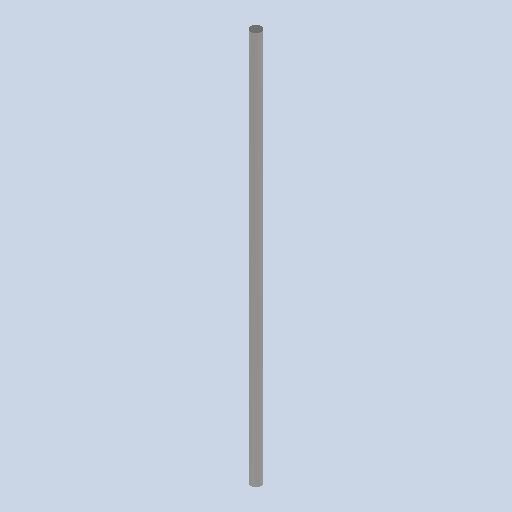
# Autodesk Inventor part: Axis
Saved by Autodesk Inventor 2023 (Build 270158000, 158)
## iProperties
Created: 2023-02-18
Part Number: Axis
Material: Stainless Steel
Document SubType Name: Modeling
Designer: phill
Density: 8 g/cm^3
Appearance: Semi-Polished
Author: phill
Autodesk Inventor part; units mm, degrees
ref_plane "YZ Plane" through (0, 0, 0) normal (1, 0, 0) x (0, 1, 0)
ref_plane "XZ Plane" through (0, 0, 0) normal (0, 1, 0) x (-1, 0, 0)
ref_plane "XY Plane" through (0, 0, 0) normal (0, 0, 1) x (1, 0, 0)
sketch "Sketch1" plane through (0, 0, 0) normal (0, 1, 0) x (-1, 0, 0)
  circle A0 centre (0, -107) radius 0.5
  circle A1 centre (0, -107) radius 1.5 projected
  arc A2 (5.6174, 110) -> (3.5, -110) centre (11433.5, -110) ccw projected
  line L0 (3.5, -110) -> (-3.5, -110) projected
  arc A3 (-3.5, -110) -> (-5.6174, 110) centre (-11433.5, -110) ccw projected
  line L1 (-5.6174, 110) -> (-3, 110) projected
  line L2 (3, 80) -> (3, 110) projected
  line L3 (3, 110) -> (5.6174, 110) projected
  line L4 (-3, 110) -> (-3, 80) projected
  line L5 (-3, 80) -> (3, 80) projected
  point P0 (0, 0)
  dimension "d0" = 1
  constraints: 1 centre point, 1 coincident
  measures "d0" diameter of A0
extrude "Extrusion1" add sketch "Sketch1" along normal blind 34 and the other way blind 2 contours A0
body "Solid1"
